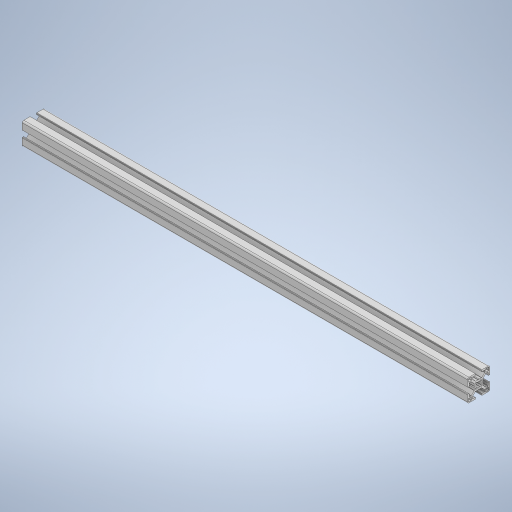
# Autodesk Inventor part: Az_rot_3030_with_holes
Saved by Autodesk Inventor 2024 (Build 280153000, 153)
## iProperties
Created: 2025-12-09
Part Number: Az_rot_3030_with_holes
Material: Generic
Document SubType Name: Modeling
Designer: schar
Density: 1 g/cm^3
Appearance: Default
Author: schar
Autodesk Inventor part; units mm, degrees
ref_plane "YZ Plane" through (0, 0, 0) normal (1, 0, 0) x (0, 1, 0)
ref_plane "XZ Plane" through (0, 0, 0) normal (0, 1, 0) x (-1, 0, 0)
ref_plane "XY Plane" through (0, 0, 0) normal (0, 0, 1) x (1, 0, 0)
sketch "Sketch1" plane through (0, 0, 0) normal (1, 0, 0) x (0, 1, 0)
  arc A0 (9.5, 9.88) -> (9.88, 9.5) centre (9.88, 9.88) ccw
  line L0 (9.88, 9.5) -> (13.3189, 9.5)
  arc A1 (13.3189, 9.5) -> (13.6999, 9.881) centre (13.3189, 9.881) ccw
  line L1 (13.6999, 9.881) -> (13.6999, 12.6999)
  arc A2 (13.6999, 12.6999) -> (12.6999, 13.6999) centre (12.6999, 12.6999) ccw
  line L2 (12.6999, 13.6999) -> (9.881, 13.6999)
  arc A3 (9.881, 13.6999) -> (9.5, 13.3189) centre (9.881, 13.3189) ccw
  line L3 (9.5, 13.3189) -> (9.5, 9.88)
  arc A4 (2.4733, -3.9799) -> (3.9799, -2.4733) centre (3.1422, -3.1422) ccw
  line L4 (3.9799, -2.4733) -> (3.1981, -1.4942)
  arc A5 (3.1981, -1.4942) -> (3.1981, 1.4942) centre (0, 0) ccw
  line L5 (3.1981, 1.4942) -> (3.9799, 2.4733)
  arc A6 (3.9799, 2.4733) -> (2.4733, 3.9799) centre (3.1422, 3.1422) ccw
  line L6 (2.4733, 3.9799) -> (1.4942, 3.1981)
  arc A7 (1.4942, 3.1981) -> (-1.4942, 3.1981) centre (0, 0) ccw
  line L7 (-1.4942, 3.1981) -> (-2.4733, 3.9799)
  arc A8 (-2.4733, 3.9799) -> (-3.9799, 2.4733) centre (-3.1422, 3.1422) ccw
  line L8 (-3.9799, 2.4733) -> (-3.1981, 1.4942)
  arc A9 (-3.1981, 1.4942) -> (-3.1981, -1.4942) centre (0, 0) ccw
  line L9 (-3.1981, -1.4942) -> (-3.9799, -2.4733)
  arc A10 (-3.9799, -2.4733) -> (-2.4733, -3.9799) centre (-3.1422, -3.1422) ccw
  line L10 (-2.4733, -3.9799) -> (-1.4942, -3.1981)
  arc A11 (-1.4942, -3.1981) -> (1.4942, -3.1981) centre (0, 0) ccw
  line L11 (1.4942, -3.1981) -> (2.4733, -3.9799)
  arc A12 (12.6999, -13.6999) -> (13.6999, -12.6999) centre (12.6999, -12.6999) ccw
  line L12 (13.6999, -12.6999) -> (13.6999, -9.881)
  arc A13 (13.6999, -9.881) -> (13.3189, -9.5) centre (13.3189, -9.881) ccw
  line L13 (13.3189, -9.5) -> (9.88, -9.5)
  arc A14 (9.88, -9.5) -> (9.5, -9.88) centre (9.88, -9.88) ccw
  line L14 (9.5, -9.88) -> (9.5, -13.3189)
  arc A15 (9.5, -13.3189) -> (9.881, -13.6999) centre (9.881, -13.3189) ccw
  line L15 (9.881, -13.6999) -> (12.6999, -13.6999)
  line L16 (14.4999, -4) -> (13.2425, -4)
  arc A16 (14.9999, -4.5) -> (14.4999, -4) centre (14.4999, -4.5) ccw
  line L17 (14.9999, -12.9999) -> (14.9999, -4.5)
  arc A17 (12.9999, -14.9999) -> (14.9999, -12.9999) centre (12.9999, -12.9999) ccw
  line L18 (4.5, -14.9999) -> (12.9999, -14.9999)
  arc A18 (4, -14.4999) -> (4.5, -14.9999) centre (4.5, -14.4999) ccw
  line L19 (4, -13.2425) -> (4, -14.4999)
  arc A19 (4.5, -12.7425) -> (4, -13.2425) centre (4.5, -13.2425) ccw
  line L20 (7.7325, -12.7425) -> (4.5, -12.7425)
  arc A20 (7.7325, -12.7425) -> (8.25, -12.2428) centre (7.75, -12.2428) ccw
  line L21 (8.25, -10.2602) -> (8.25, -12.2428)
  arc A21 (8.25, -10.2602) -> (8.1035, -9.9066) centre (7.75, -10.2602) ccw
  line L22 (4.178, -5.9811) -> (8.1035, -9.9066)
  arc A22 (4.178, -5.9811) -> (3.8245, -5.8347) centre (3.8245, -6.3347) ccw
  line L23 (0.95, -5.8347) -> (3.8245, -5.8347)
  line L24 (0, -5.3247) -> (0.95, -5.8347)
  line L25 (-0.95, -5.8347) -> (0, -5.3247)
  line L26 (-3.8245, -5.8347) -> (-0.95, -5.8347)
  arc A23 (-3.8245, -5.8347) -> (-4.178, -5.9811) centre (-3.8245, -6.3347) ccw
  line L27 (-8.1035, -9.9066) -> (-4.178, -5.9811)
  arc A24 (-8.1035, -9.9066) -> (-8.25, -10.2602) centre (-7.75, -10.2602) ccw
  line L28 (-8.25, -12.2428) -> (-8.25, -10.2602)
  arc A25 (-8.25, -12.2428) -> (-7.7325, -12.7425) centre (-7.75, -12.2428) ccw
  line L29 (-4.5, -12.7425) -> (-7.7325, -12.7425)
  arc A26 (-4, -13.2425) -> (-4.5, -12.7425) centre (-4.5, -13.2425) ccw
  line L30 (-4, -14.4999) -> (-4, -13.2425)
  arc A27 (-4.5, -14.9999) -> (-4, -14.4999) centre (-4.5, -14.4999) ccw
  line L31 (-12.9999, -14.9999) -> (-4.5, -14.9999)
  arc A28 (-14.9999, -12.9999) -> (-12.9999, -14.9999) centre (-12.9999, -12.9999) ccw
  line L32 (-14.9999, -4.5) -> (-14.9999, -12.9999)
  arc A29 (-14.4999, -4) -> (-14.9999, -4.5) centre (-14.4999, -4.5) ccw
  line L33 (-13.2425, -4) -> (-14.4999, -4)
  arc A30 (-12.7425, -4.5) -> (-13.2425, -4) centre (-13.2425, -4.5) ccw
  line L34 (-12.7425, -7.7325) -> (-12.7425, -4.5)
  arc A31 (-12.7425, -7.7325) -> (-12.2428, -8.25) centre (-12.2428, -7.75) ccw
  line L35 (-10.2602, -8.25) -> (-12.2428, -8.25)
  arc A32 (-10.2602, -8.25) -> (-9.9066, -8.1035) centre (-10.2602, -7.75) ccw
  line L36 (-5.9811, -4.178) -> (-9.9066, -8.1035)
  arc A33 (-5.9811, -4.178) -> (-5.8347, -3.8245) centre (-6.3347, -3.8245) ccw
  line L37 (-5.8347, -1.0125) -> (-5.8347, -3.8245)
  line L38 (-5.3247, -0.0625) -> (-5.8347, -1.0125)
  line L39 (-5.8347, 0.8875) -> (-5.3247, -0.0625)
  line L40 (-5.8347, 3.8245) -> (-5.8347, 0.8875)
  arc A34 (-5.8347, 3.8245) -> (-5.9811, 4.178) centre (-6.3347, 3.8245) ccw
  line L41 (-9.9066, 8.1035) -> (-5.9811, 4.178)
  arc A35 (-9.9066, 8.1035) -> (-10.2602, 8.25) centre (-10.2602, 7.75) ccw
  line L42 (-12.2428, 8.25) -> (-10.2602, 8.25)
  arc A36 (-12.2428, 8.25) -> (-12.7425, 7.7325) centre (-12.2428, 7.75) ccw
  line L43 (-12.7425, 4.5) -> (-12.7425, 7.7325)
  arc A37 (-13.2425, 4) -> (-12.7425, 4.5) centre (-13.2425, 4.5) ccw
  line L44 (-14.4999, 4) -> (-13.2425, 4)
  arc A38 (-14.9999, 4.5) -> (-14.4999, 4) centre (-14.4999, 4.5) ccw
  line L45 (-14.9999, 12.9999) -> (-14.9999, 4.5)
  arc A39 (-12.9999, 14.9999) -> (-14.9999, 12.9999) centre (-12.9999, 12.9999) ccw
  line L46 (-4.5, 14.9999) -> (-12.9999, 14.9999)
  arc A40 (-4, 14.4999) -> (-4.5, 14.9999) centre (-4.5, 14.4999) ccw
  line L47 (-4, 13.2425) -> (-4, 14.4999)
  arc A41 (-4.5, 12.7425) -> (-4, 13.2425) centre (-4.5, 13.2425) ccw
  line L48 (-7.7325, 12.7425) -> (-4.5, 12.7425)
  arc A42 (-7.7325, 12.7425) -> (-8.25, 12.2428) centre (-7.75, 12.2428) ccw
  line L49 (-8.25, 10.2602) -> (-8.25, 12.2428)
  arc A43 (-8.25, 10.2602) -> (-8.1035, 9.9066) centre (-7.75, 10.2602) ccw
  line L50 (-4.178, 5.9811) -> (-8.1035, 9.9066)
  arc A44 (-4.178, 5.9811) -> (-3.8245, 5.8347) centre (-3.8245, 6.3347) ccw
  line L51 (-0.95, 5.8347) -> (-3.8245, 5.8347)
  line L52 (0, 5.3247) -> (-0.95, 5.8347)
  line L53 (0.95, 5.8347) -> (0, 5.3247)
  line L54 (3.8245, 5.8347) -> (0.95, 5.8347)
  arc A45 (3.8245, 5.8347) -> (4.178, 5.9811) centre (3.8245, 6.3347) ccw
  line L55 (8.1035, 9.9066) -> (4.178, 5.9811)
  arc A46 (8.1035, 9.9066) -> (8.25, 10.2602) centre (7.75, 10.2602) ccw
  line L56 (8.25, 12.2428) -> (8.25, 10.2602)
  arc A47 (8.25, 12.2428) -> (7.7325, 12.7425) centre (7.75, 12.2428) ccw
  line L57 (4.5, 12.7425) -> (7.7325, 12.7425)
  arc A48 (4, 13.2425) -> (4.5, 12.7425) centre (4.5, 13.2425) ccw
  line L58 (4, 14.4999) -> (4, 13.2425)
  arc A49 (4.5, 14.9999) -> (4, 14.4999) centre (4.5, 14.4999) ccw
  line L59 (12.9999, 14.9999) -> (4.5, 14.9999)
  arc A50 (14.9999, 12.9999) -> (12.9999, 14.9999) centre (12.9999, 12.9999) ccw
  line L60 (14.9999, 4.5) -> (14.9999, 12.9999)
  arc A51 (14.4999, 4) -> (14.9999, 4.5) centre (14.4999, 4.5) ccw
  line L61 (13.2425, 4) -> (14.4999, 4)
  arc A52 (12.7425, 4.5) -> (13.2425, 4) centre (13.2425, 4.5) ccw
  line L62 (12.7425, 7.7325) -> (12.7425, 4.5)
  arc A53 (12.7425, 7.7325) -> (12.2428, 8.25) centre (12.2428, 7.75) ccw
  line L63 (10.2602, 8.25) -> (12.2428, 8.25)
  arc A54 (10.2602, 8.25) -> (9.9066, 8.1035) centre (10.2602, 7.75) ccw
  line L64 (5.9811, 4.178) -> (9.9066, 8.1035)
  arc A55 (5.9811, 4.178) -> (5.8347, 3.8245) centre (6.3347, 3.8245) ccw
  line L65 (5.8347, 0.8875) -> (5.8347, 3.8245)
  line L66 (5.3247, -0.0625) -> (5.8347, 0.8875)
  line L67 (5.8347, -1.0125) -> (5.3247, -0.0625)
  line L68 (5.8347, -3.8245) -> (5.8347, -1.0125)
  arc A56 (5.8347, -3.8245) -> (5.9811, -4.178) centre (6.3347, -3.8245) ccw
  line L69 (9.9066, -8.1035) -> (5.9811, -4.178)
  arc A57 (9.9066, -8.1035) -> (10.2602, -8.25) centre (10.2602, -7.75) ccw
  line L70 (12.2428, -8.25) -> (10.2602, -8.25)
  arc A58 (12.2428, -8.25) -> (12.7425, -7.7325) centre (12.2428, -7.75) ccw
  line L71 (12.7425, -4.5) -> (12.7425, -7.7325)
  arc A59 (13.2425, -4) -> (12.7425, -4.5) centre (13.2425, -4.5) ccw
  arc A60 (-13.6999, -12.6999) -> (-12.6999, -13.6999) centre (-12.6999, -12.6999) ccw
  line L72 (-12.6999, -13.6999) -> (-9.881, -13.6999)
  arc A61 (-9.881, -13.6999) -> (-9.5, -13.3189) centre (-9.881, -13.3189) ccw
  line L73 (-9.5, -13.3189) -> (-9.5, -9.88)
  arc A62 (-9.5, -9.88) -> (-9.88, -9.5) centre (-9.88, -9.88) ccw
  line L74 (-9.88, -9.5) -> (-13.3189, -9.5)
  arc A63 (-13.3189, -9.5) -> (-13.6999, -9.881) centre (-13.3189, -9.881) ccw
  line L75 (-13.6999, -9.881) -> (-13.6999, -12.6999)
  arc A64 (-12.6999, 13.6999) -> (-13.6999, 12.6999) centre (-12.6999, 12.6999) ccw
  line L76 (-13.6999, 12.6999) -> (-13.6999, 9.881)
  arc A65 (-13.6999, 9.881) -> (-13.3189, 9.5) centre (-13.3189, 9.881) ccw
  line L77 (-13.3189, 9.5) -> (-9.88, 9.5)
  arc A66 (-9.88, 9.5) -> (-9.5, 9.88) centre (-9.88, 9.88) ccw
  line L78 (-9.5, 9.88) -> (-9.5, 13.3189)
  arc A67 (-9.5, 13.3189) -> (-9.881, 13.6999) centre (-9.881, 13.3189) ccw
  line L79 (-9.881, 13.6999) -> (-12.6999, 13.6999)
  point P0 (4.5, -12.7425)
  point P1 (4, -14.4999)
  point P2 (12.9999, -14.9999)
  point P3 (14.9999, -4.5)
  point P4 (12.7425, -7.7325)
  point P5 (10.2602, -8.25)
  point P6 (5.9811, -4.178)
  point P7 (9.9066, 8.1035)
  point P8 (12.2428, 8.25)
  point P9 (14.4999, 4)
  point P10 (14.9999, 12.9999)
  point P11 (4.5, 14.9999)
  point P12 (4, 13.2425)
  point P13 (7.7325, 12.7425)
  point P14 (8.25, 10.2602)
  point P15 (4.178, 5.9811)
  point P16 (-3.8245, 5.8347)
  point P17 (-8.1035, 9.9066)
  point P18 (-8.25, 12.2428)
  point P19 (-4.5, 12.7425)
  point P20 (-4, 14.4999)
  point P21 (-12.9999, 14.9999)
  point P22 (-14.9999, 4.5)
  point P23 (-13.2425, 4)
  point P24 (-12.7425, 7.7325)
  point P25 (-10.2602, 8.25)
  point P26 (-5.9811, 4.178)
  point P27 (-5.8347, -3.8245)
  point P28 (-9.9066, -8.1035)
  point P29 (-12.2428, -8.25)
  point P30 (-12.7425, -4.5)
  point P31 (-14.9999, -12.9999)
  point P32 (-4.5, -14.9999)
  point P33 (-4, -13.2425)
  point P34 (-7.7325, -12.7425)
  point P35 (-8.25, -10.2602)
  point P36 (-4.178, -5.9811)
  point P37 (3.8245, -5.8347)
  point P38 (8.1035, -9.9066)
  point P39 (8.25, -12.2428)
  point P40 (-12.6999, 13.6999)
  point P41 (-9.5, 9.88)
  point P42 (-13.3189, 9.5)
  point P43 (-13.6999, 12.6999)
  point P44 (-13.6999, -12.6999)
  point P45 (-13.6999, -9.881)
  point P46 (-9.5, -13.3189)
  point P47 (-12.6999, -13.6999)
  point P48 (12.6999, -13.6999)
  point P49 (9.881, -13.6999)
  point P50 (9.5, -9.88)
  point P51 (13.3189, -9.5)
  point P52 (13.6999, -12.6999)
  point P53 (2.4733, -3.9799)
  point P54 (1.4942, -3.1981)
  point P55 (-2.4733, -3.9799)
  point P56 (-3.1981, -1.4942)
  point P57 (-3.9799, 2.4733)
  point P58 (-1.4942, 3.1981)
  point P59 (2.4733, 3.9799)
  point P60 (3.1981, 1.4942)
  point P61 (3.9799, -2.4733)
  point P62 (9.5, 9.88)
  point P63 (9.88, 9.5)
  constraints: 160 end point, 136 point on circle, 68 centre point
extrude "Extrusion1" add sketch "Sketch1" along normal blind 600
ref_plane "Work Plane1" through (0, 4.5, 14.9999) normal (0, 0, 1) x (1, 0, 0)
sketch "Sketch3" plane through (0, 4.5, 14.9999) normal (0, 0, 1) x (1, 0, 0)
  line L0 (0, 10.4999) -> (10, 10.4999)
  line L1 (0, 10.4999) -> (600, 10.4999) projected
  line L2 (10, 10.4999) -> (10, -4.5)
  line L3 (10, 10.4999) -> (48, 10.4999)
  line L4 (48, 10.4999) -> (48, -4.5)
  line L5 (0, -4.5) -> (600, -4.5) projected
  line L6 (48, 10.4999) -> (86, 10.4999)
  line L7 (86, 10.4999) -> (86, -4.5)
  circle A0 centre (10, -4.5) radius 3
  circle A1 centre (48, -4.5) radius 3
  circle A2 centre (86, -4.5) radius 3
  dimension "d3" = 10
  dimension "d4" = 38
  dimension "d5" = 38
  dimension "d6" = 6
  dimension "d7" = 6
  dimension "d8" = 6
  constraints: 12 end point, 4 point on line, 3 centre point, 3 coincident, 3 perpendicular
  measures "d3" distance of L0.start L0.end
  measures "d4" distance of L0.end L3.end
  measures "d5" distance of L3.end L6.end
  measures "d6" diameter of A0
  measures "d7" diameter of A1
  measures "d8" diameter of A2
extrude "Extrusion2" cut sketch "Sketch3" against normal blind 30 contours A0 L5 L2 | L2 L5 A0 | A1 L5 L4 | L4 L5 A1 | L5 A0 | A2 L5 L7 | L7 L5 A2 | L5 A1 | L5 A2
body "Solid1"
